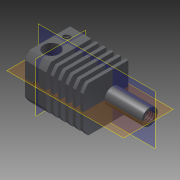
# Autodesk Inventor part: D-045
Saved by Autodesk Inventor 2015 (Build 190159000, 159)
## iProperties
Company: MARCHA TECHNOLOGY SL
Created: 2014-05-13
Part Number: D-045
Document SubType Name: Modeling
Designer: O.Martin
Density: 1 g/cm^3
Project: HOTEND PROTOTIPO
Description: HOTEND ONE BODY CUERPO
Stock Number: 28658
Material: Generic
Appearance: Gray
Author: O.Martin
Autodesk Inventor part; units mm, degrees
ref_plane "YZ Plane" through (0, 0, 0) normal (1, 0, 0) x (0, 1, 0)
sketch "Boceto1" plane through (0, 0, 0) normal (0, 0, 1) x (1, 0, 0)
  line L0 (0, 0) -> (48, 0)
  line L1 (48, 0) -> (48, -1.5566)
  line L2 (48, -1.5566) -> (45.5, -3)
  line L3 (45.5, -3) -> (26, -3)
  line L4 (26, -3) -> (26, -12.5)
  line L5 (4, -12.5) -> (4, -4)
  line L6 (4, -4) -> (3.6, -4)
  line L7 (3.6, -4) -> (0, -0.4)
  line L8 (0, -0.4) -> (0, 0)
  line L9 (15, -2) -> (15, -1)
  line L10 (15, -1) -> (1.3, -1)
  line L11 (1.3, -1) -> (0.5, -0.2)
  line L12 (0.5, -0.2) -> (0, -0.2)
  circle A0 centre (8, -5) radius 3
  line L13 (12, -12.5) -> (12, -4)
  line L14 (12, -4) -> (13.6, -4)
  line L15 (15, -2) -> (33, -2)
  line L16 (47.15, -1) -> (40, -1)
  line L17 (47.15, -1) -> (48, -1.4907)
  line L18 (4, -12.5) -> (12, -12.5)
  line L19 (13.6, -4) -> (13.6, -12.5)
  line L20 (13.6, -12.5) -> (26, -12.5)
  line L21 (14.8, -12.5) -> (16.4, -12.5)
  line L22 (16.4, -12.5) -> (16.4, -4)
  line L23 (16.4, -4) -> (14.8, -4)
  line L24 (14.8, -4) -> (14.8, -12.5)
  line L25 (17.6, -12.5) -> (19.2, -12.5)
  line L26 (19.2, -12.5) -> (19.2, -4)
  line L27 (19.2, -4) -> (17.6, -4)
  line L28 (17.6, -4) -> (17.6, -12.5)
  line L29 (20.4, -12.5) -> (22, -12.5)
  line L30 (22, -12.5) -> (22, -4)
  line L31 (22, -4) -> (20.4, -4)
  line L32 (20.4, -4) -> (20.4, -12.5)
  line L33 (33, -2) -> (33, -2)
  line L34 (33, -2) -> (34, -2)
  line L35 (34, -2) -> (34, -2)
  line L36 (34, -2) -> (40, -2)
  line L37 (40, -2) -> (40, -3)
  line L38 (23.2, -12.5) -> (24.8, -12.5)
  line L39 (24.8, -12.5) -> (24.8, -4)
  line L40 (24.8, -4) -> (23.2, -4)
  line L41 (23.2, -4) -> (23.2, -12.5)
  line L42 (26, -12.5) -> (27.6, -12.5)
  line L43 (27.6, -12.5) -> (27.6, -4)
  line L44 (27.6, -4) -> (26, -4)
  line L45 (26, -4) -> (26, -12.5)
  line L46 (1.3, -1) -> (0.6, -1) construction
  line L47 (1.3, -1) -> (0.95, -1.35) construction
  dimension "d0" = 48
  dimension "d1" = 0.8
  dimension "d2" = 4
  dimension "d5" = 6
  dimension "d6" = 2.5
  dimension "d7" = 30
  dimension "d8" = 45
  dimension "d9" = 8
  dimension "d10" = 0.4
  dimension "d11" = 0.5
  dimension "d12" = 2
  dimension "d13" = 45
  dimension "d15" = 11
  dimension "d16" = 5
  dimension "d17" = 6
  dimension "d18" = 4
  dimension "d19" = 8
  dimension "d21" = 4
  dimension "d36" = 4
  dimension "d37" = 2
  dimension "d39" = 0.85
  dimension "d40" = 30
  dimension "d49" = 25
  dimension "d50" = 25
  dimension "d51" = 22
  dimension "d52" = 1.6
  dimension "d53" = 1.2
  dimension "d55" = 1.2
  dimension "d57" = 1.6
  dimension "d58" = 1.2
  dimension "d64" = 8
  dimension "d65" = 6
  dimension "d66" = 1
  dimension "d67" = 4
  dimension "d68" = 4
  dimension "d88" = 1.2
  dimension "d89" = 1.2
  dimension "d102" = 1.6
  dimension "d103" = 0.495
  dimension "d104" = 0.7
  constraints: 96 end point, 20 parallel, 14 perpendicular, 9 point on line, 7 equal length, 7 horizontal, 1 centre point, 1 coincident, 1 collinear, 1 horizontal alignment, 1 midpoint
  measures "d0" distance of L0.start L0.end
  measures "d1" diameter of L7.end L0
  measures "d2" distance between parallel lines of L5 L8
  measures "d5" diameter of L3 L0
  measures "d6" horizontal distance of L1.end L2.end
  measures "d7" angle of L2 L3
  measures "d8" angle of L6 L7
  measures "d9" diameter of L6 L0
  measures "d10" diameter of L12 L0
  measures "d11" distance of L11.end L12.end
  measures "d12" diameter of L10 L0
  measures "d13" angle of L0 L11
  measures "d15" distance between parallel lines of L5 L9
  measures "d16" vertical distance of L0.start A0.centre
  measures "d17" diameter of A0
  measures "d18" distance from line of A0.centre L5
  measures "d19" distance between parallel lines of L13 L5
  measures "d21" distance from line of L0.start L14
  measures "d36" diameter of L15 L0
  measures "d37" diameter of L16 L0
  measures "d39" horizontal distance of L16.start L17.end
  measures "d40" angle of L16 L17
  measures "d49" diameter of L18 L0
  measures "d50" diameter of L20 L0
  measures "d51" distance between parallel lines of L5 L4
  measures "d52" distance between parallel lines of L13 L19
  measures "d53" distance between parallel lines of L24 L19
  measures "d55" distance between parallel lines of L28 L22
  measures "d57" distance between parallel lines of L26 L28
  measures "d58" distance between parallel lines of L32 L26
  measures "d64" distance between parallel lines of L1 L37
  measures "d65" distance of L35.end L36.end
  measures "d66" distance of L33.end L34.end
  measures "d67" diameter of L34 L0
  measures "d68" diameter of L36 L0
  measures "d88" distance between parallel lines of L41 L30
  measures "d89" distance between parallel lines of L45 L39
  measures "d102" distance of L22.end L23.end
  measures "d103" distance of L10.end L47.end
  measures "d104" distance of L10.end L46.end
revolve "Revolución1" add sketch "Boceto1" angle 360 about axis through (0, 0, 0) along (1, 0, 0) contours L12 L11 L10 L9 L15 L34 L36 L37 L3 L4 L20 L39 L40 L41 L30 L31 L32 L26 L27 L28 L22 L23 L24 L19 L14 L13 L18 L5 L6 L7 L8 | A0
sketch "Boceto2" plane through (4, 0, 0) normal (-1, 0, 0) x (0, 0, 1)
  circle A0 centre (0, 0) radius 4 projected
  line L0 (-8.5, 6) -> (8.5, 6)
  line L1 (8.5, 6) -> (8.5, -11)
  line L2 (8.5, -11) -> (-8.5, -11)
  line L3 (-8.5, -11) -> (-8.5, 6)
  dimension "d27" = 17
  dimension "d28" = 17
  dimension "d29" = 8.5
  dimension "d30" = 6
  constraints: 8 end point, 2 parallel, 1 horizontal, 1 perpendicular
  measures "d27" distance of L0.start L0.end
  measures "d28" distance of L0.end L1.end
  measures "d29" distance from line of A0.centre L3
  measures "d30" distance from line of A0.centre L0
extrude "Extrusión1" cut sketch "Boceto2" along normal through all both and the other way through all contours A0 | L0 L1 L2 L3 keep common part
extrude "Extrusión2" cut sketch "Boceto1" along normal through all both and the other way through all contours A0
sketch "Boceto3" plane through (4, -11, 8.5) normal (0, 0, 1) x (1, 0, 0)
  arc A0 (7, 2) -> (7, 2) centre (4, 6) ccw
  circle A1 centre (4, 6) radius 3 projected
  line L0 (0, 17) -> (0, 1.8348) projected
  point P0 (8, 2)
  point P1 (2.75, 13)
  dimension "d100" = 2.75
  dimension "d101" = 7
  constraints: 1 coincident, 4 other
  measures "d100" distance from line of point (2.75, 13) L0
  measures "d101" vertical distance of point (4, 6) point (2.75, 13)
hole "Agujero1" at (6.75, 2, 8.5) direction (0, 0, -1) diameter 2.459 depth 6 tip angle 118 thread size "M3x0.5" class "6H" standard "ISO Metric profile"
hole "Agujero2" at (40, 0, 0) direction (-1, 0, 0) diameter 4.134 depth 6.5 thread size "M5x0.8" class "6H" standard "ISO Metric profile"
sketch "Boceto4" plane through (4, -11, -5.9372) normal (0, -1, 0) x (1, 0, 0)
  line L0 (0, 11.8743) -> (0, 0) projected
  line L1 (7, -2.5628) -> (1, -2.5628) projected
  point P0 (4, 5.9372)
  point P1 (0, 5.9372)
  point P2 (0, 13.8852)
  point P3 (0, -3.1148)
  point P4 (4.7082, -5.1459)
  point P5 (2.2918, -5.1459)
  point P6 (1, -2.5628)
  point P7 (4, -2.5628)
  constraints: 1 horizontal alignment, 1 midpoint, 1 vertical alignment, 2 other
hole "Agujero4" at (8, -11, 0) direction (0, 1, 0) diameter 2.459 end up to face face through (8, -5, 0) facing (0, 0, 1) round with radius 3 far side yes thread size "M3x0.5" class "6H" standard "ISO Metric profile"
ref_plane "Plano de trabajo1" through (9, -9.1652, 8.5) normal (-1, 0, 0) x (0, 0, 1)
mirror "Simetría1" about plane through (0, 0, 0) normal (0, 0, 1) of "Agujero1"
equation "\"d29\" = 0.5 * d27"
equation "\"d55\" = d53"
equation "\"d58\" = d55"
equation "\"d88\" = d58"
equation "\"d89\" = d88"
body "Solid1"
